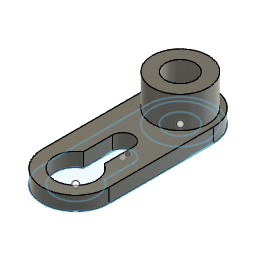
Semana2_Desafio3 (Autodesk Fusion 360 design; units mm, degrees)
Autodesk Fusion 360 part; units mm, degrees
sketch "Sketch1" plane through (0, 0, 0) normal (0, 1, 0) x (1, 0, 0)
  line L0 (-95, 150) -> (-95, -150)
  line L1 (95, -150) -> (95, 150)
  circle A0 centre (0, 150) radius 80
  circle A1 centre (0, 150) radius 42.5
  line L2 (-30, -15) -> (-30, -98.0385)
  line L3 (30, -98.0385) -> (30, -15)
  arc A2 (-95, -150) -> (95, -150) centre (0, -150) ccw
  arc A3 (30, -15) -> (-30, -15) centre (0, -15) ccw
  arc A4 (95, 150) -> (-95, 150) centre (0, 150) ccw
  arc A5 (-30, -98.0385) -> (30, -98.0385) centre (0, -150) ccw
  dimension "d1" = 190
  dimension "d2" = 300
  dimension "d3" = 160
  dimension "d4" = 85
  dimension "d9" = 120
  dimension "d11" = 30
  dimension "d12" = 60
  constraint parallel L0 L1
  constraint concentric A0 A4
  constraint concentric A1 A4
  constraint vertical L2
  constraint vertical L3
  measures "d1" distance of L0.end L1.start
  measures "d2" distance of L0.start L0.end
  measures "d3" diameter of A0
  measures "d4" diameter of A1
  measures "d9" diameter of A5
  measures "d11" distance of L3.end A3.centre
  measures "d12" distance of L3.end L2.start
extrude "Extrude1" add sketch "Sketch1" along normal blind 130 contours A0
extrude "Extrude2" add sketch "Sketch1" along normal blind 40
